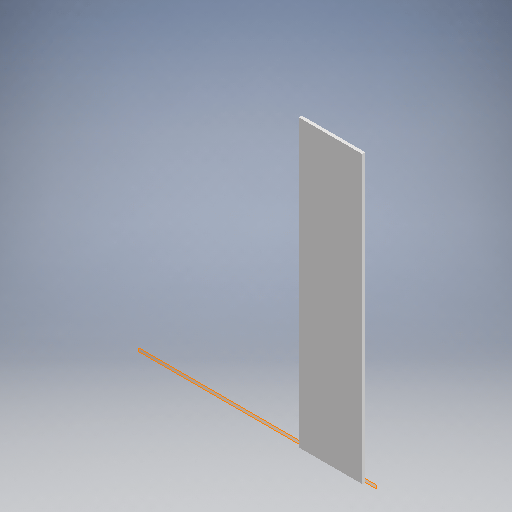
# Autodesk Inventor part: RIGHT B THE DOOR
Saved by Autodesk Inventor 2025.2 (Build 292293000, 293)
## iProperties
Created: 2025-01-27
Part Number: RIGHT B THE DOOR
Material: Generic
Document SubType Name: Modeling
Designer: Anna
Density: 1 g/cm^3
Appearance: Default
Author: Anna
Autodesk Inventor part; units mm, degrees
ref_plane "YZ Plane" through (0, 0, 0) normal (1, 0, 0) x (0, 1, 0)
ref_plane "XZ Plane" through (0, 0, 0) normal (0, 1, 0) x (-1, 0, 0)
ref_plane "XY Plane" through (0, 0, 0) normal (0, 0, 1) x (1, 0, 0)
ref_plane "Work Plane1" through (0, 0, 0) normal (0, 0, 1) x (1, 0, 0)
sketch "Sketch1" plane through (0, 0, 0) normal (0, 0, 1) x (1, 0, 0)
  line L0 (1803.4, 2387.6) -> (1803.4, 0) projected
  line L1 (1803.4, 0) -> (1270, 0)
  line L2 (1270, 0) -> (1270, 2387.6)
  line L3 (1270, 2387.6) -> (1803.4, 2387.6)
  point P0 (0, 0)
  dimension "d0" = 533.4
  dimension "d1" = 2387.6
  constraints: 6 end point, 1 horizontal, 1 perpendicular
  measures "d0" distance of L0.end L1.end
  measures "d1" distance of L1.end L2.end
extrude "Extrusion1" add sketch "Sketch1" along normal blind 25.4
body "Solid1"
